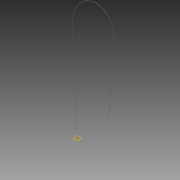
# Autodesk Inventor part: M2Thread
Saved by Autodesk Inventor 2012 SP2 (Build 160219200, 219)
## iProperties
Created: 2013-07-20
Part Number: M2Thread
Material: Default
Document SubType Name: Modeling
Designer: 1
Density: 1 g/cm^3
Author: 1
Autodesk Inventor part; units mm, degrees
ref_plane "YZ Plane" through (0, 0, 0) normal (1, 0, 0) x (0, 1, 0)
ref_plane "XZ Plane" through (0, 0, 0) normal (0, 1, 0) x (-1, 0, 0)
ref_plane "XY Plane" through (0, 0, 0) normal (0, 0, 1) x (1, 0, 0)
sketch "Sketch1" plane through (0, 0, 0) normal (0, 0, 1) x (1, 0, 0)
  line L0 (-62.8016, -575) -> (-6.8016, -575) projected
  circle A0 centre (39.9984, 76.5) radius 74.8 construction
  line L1 (-34.8016, -375) -> (-34.8016, 76.5)
  line L2 (114.7984, 76.5) -> (114.7984, -173.5)
  arc A1 (114.7984, 76.5) -> (-34.8016, 76.5) centre (39.9984, 76.5) ccw
  dimension "d0" = 200
  dimension "d6" = 250
  constraints: 4 end point, 4 point on circle, 2 tangent, 1 centre point, 1 coincident, 1 parallel, 1 perpendicular
  measures "d0" distance from line of L0 L1.start
  measures "d6" distance of L2.start L2.end
ref_plane "Work Plane1" through (-34.8016, -375, 0) normal (0, 1, 0) x (-1, 0, 0)
sketch "Sketch2" plane through (-34.8016, -375, 0) normal (0, 1, 0) x (-1, 0, 0)
  circle A0 centre (0, 0) radius 0.4
  point P0 (-34.8016, 0)
  dimension "d2" = 0.8
  dimension "d3" = 34.8016
  constraints: 1 centre point
  measures "d2" diameter of A0
  measures "d3" distance of A0.centre point (-34.802, 0)
sweep "Sweep2" add profiles "Sketch2" path "Sketch1" path curves L1 A1 L2
body "Solid2"
